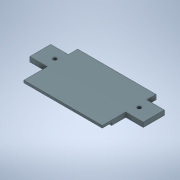
# Autodesk Inventor part: WeightBack
Saved by Autodesk Inventor 2021 (Build 250183000, 183)
## iProperties
Created: 2022-04-12
Part Number: WeightBack
Material: Lead
Document SubType Name: Modeling
Designer: ermoz
Density: 11.34 g/cm^3
Appearance: Lead
Author: ermoz
Autodesk Inventor part; units mm, degrees
ref_plane "YZ Plane" through (0, 0, 0) normal (1, 0, 0) x (0, 1, 0)
ref_plane "XZ Plane" through (0, 0, 0) normal (0, 1, 0) x (-1, 0, 0)
ref_plane "XY Plane" through (0, 0, 0) normal (0, 0, 1) x (1, 0, 0)
sketch "Sketch1" plane through (0, 0, 0) normal (0, 1, 0) x (-1, 0, 0)
  line L0 (-33.5, -23) -> (33.5, -23)
  line L1 (33.5, -23) -> (33.5, 23)
  line L2 (33.5, 23) -> (-33.5, 23)
  line L3 (-33.5, 23) -> (-33.5, -23)
  line L4 (-33.5, -23) -> (33.5, 23) construction
  line L5 (33.5, -23) -> (-33.5, 23) construction
  line L6 (33.5, 3) -> (48.5, 3)
  line L7 (48.5, 3) -> (48.5, -15)
  line L8 (48.5, -15) -> (33.5, -15)
  line L9 (33.5, -15) -> (33.5, 3)
  line L10 (-33.5, 3) -> (-48.5, 3)
  line L11 (-48.5, 3) -> (-48.5, -15)
  line L12 (-48.5, -15) -> (-33.5, -15)
  line L13 (-33.5, -15) -> (-33.5, 3)
  point P0 (0, 0)
  point P1 (-33.5, 3)
  dimension "d0" = 67
  dimension "d1" = 46
  dimension "d2" = 97
  dimension "d5" = 8
  dimension "d6" = 18
  constraints: 28 end point, 6 parallel, 5 collinear, 3 horizontal, 3 perpendicular, 2 midpoint
  measures "d0" distance of L1.end L2.end
  measures "d1" distance of L0.end L1.end
  measures "d2" distance between parallel lines of L11 L7
  measures "d5" distance between parallel lines of L0 L8
  measures "d6" distance of L6.end L7.end
extrude "Extrusion1" add sketch "Sketch1" along normal blind 4
sketch "Sketch2" plane through (0, 0, 0) normal (0, -1, 0) x (1, 0, 0)
  line L0 (-33.5, 23) -> (33.5, 23) projected
  line L1 (33.5, 23) -> (33.5, 3) projected
  line L2 (-33.5, 23) -> (33.5, 23)
  line L3 (33.5, 23) -> (33.5, 15)
  line L4 (33.5, 15) -> (-33.5, 15)
  line L5 (-33.5, 15) -> (-33.5, 23)
  point P0 (0, 0)
  dimension "d7" = 8
  constraints: 8 end point, 2 parallel, 1 horizontal, 1 perpendicular, 1 point on line
  measures "d7" distance between parallel lines of L0 L4
extrude "Extrusion2" cut sketch "Sketch2" against normal blind 2
sketch "Sketch3" plane through (0, 0, 0) normal (0, -1, 0) x (1, 0, 0)
  circle A0 centre (-36, -6) radius 1.5
  circle A1 centre (36, -6) radius 1.5
  line L0 (48.5, -15) -> (33.5, -15) projected
  line L1 (48.5, 3) -> (48.5, -15) projected
  line L2 (-48.5, -15) -> (-48.5, 3) projected
  line L3 (-33.5, -15) -> (-48.5, -15) projected
  point P0 (0, 0)
  dimension "d10" = 9
  dimension "d11" = 12.5
  dimension "d12" = 12.5
  dimension "d13" = 9
  dimension "d14" = 3
  constraints: 2 centre point, 1 equal radius
  measures "d10" distance from line of L0 A1.centre
  measures "d11" distance from line of L1 A1.centre
  measures "d12" distance from line of L2 A0.centre
  measures "d13" distance from line of L3 A0.centre
  measures "d14" diameter of A1
extrude "Extrusion3" cut sketch "Sketch3" against normal through all
chamfer "Chamfer1" distance 2 angle 45 2 edges at (34.5, 0, -6) (-37.5, 0, -6)
body "Solid1"
